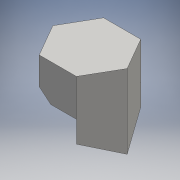
# Autodesk Inventor part: призму
Saved by Autodesk Inventor 2016 (Build 200138000, 138)
## iProperties
Created: 2016-10-05
Part Number: призму
Material: Типовые
Document SubType Name: Modeling
Designer: Student
Density: 1 g/cm^3
Appearance: По умолчанию
Author: Student
Autodesk Inventor part; units mm, degrees
ref_plane "YZ Plane" through (0, 0, 0) normal (1, 0, 0) x (0, 1, 0)
ref_plane "XZ Plane" through (0, 0, 0) normal (0, 1, 0) x (-1, 0, 0)
ref_plane "XY Plane" through (0, 0, 0) normal (0, 0, 1) x (1, 0, 0)
sketch "Эскиз1" plane through (0, 0, 0) normal (0, 0, 1) x (1, 0, 0)
  line L0 (25, 0) -> (12.5, -21.6506)
  line L1 (12.5, -21.6506) -> (-12.5, -21.6506)
  line L2 (-12.5, -21.6506) -> (-25, 0)
  line L3 (-25, 0) -> (-12.5, 21.6506)
  line L4 (-12.5, 21.6506) -> (12.5, 21.6506)
  line L5 (12.5, 21.6506) -> (25, 0)
  point P0 (0, 0)
  point P1 (0, 0)
  constraints: 12 end point, 13 other
extrude "Выдавливание1" add sketch "Эскиз1" along normal blind 50
sketch "Эскиз2" plane through (-12.5, 21.6506, 0) normal (0, 1, 0) x (1, 0, 0)
  point P0 (12.5, 0)
sketch "Эскиз3" plane through (-12.5, 21.6506, 0) normal (0, 1, 0) x (1, 0, 0)
  line L0 (-12.5, 0) -> (0, 0) projected
  line L1 (-12.5, -50) -> (-12.5, 0)
  line L2 (37.5, 0) -> (25, 0) projected
  line L3 (37.5, 0) -> (-12.5, 0)
  line L4 (37.5, 0) -> (37.5, -50) projected
  line L5 (37.5, 0) -> (37.5, -50)
  line L6 (0, -50) -> (-12.5, -50) projected
  line L7 (37.5, -50) -> (-12.5, -50)
  line L8 (-12.5, 0) -> (-12.5, -50) projected
  line L9 (25, -10.4887) -> (25, -50)
  line L10 (37.5, 0) -> (25, -10.4887)
  line L11 (7.7062, -25) -> (-12.5, -41.955)
  line L12 (7.7062, -25) -> (25, -25)
  point P0 (12.5, 0)
  constraints: 16 end point, 3 point on line, 2 collinear, 2 vertical, 1 horizontal, 1 perpendicular
extrude "Выдавливание2" cut sketch "Эскиз3" against normal blind 50 contours L0 L3 L2 L10 L9 L12 L11 L1
